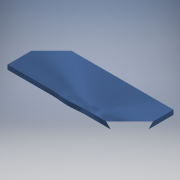
# Autodesk Inventor part: Cup_Dispenser_Slider_Cover
Saved by Autodesk Inventor 2016 (Build 200138000, 138)
## iProperties
Created: 2015-07-07
Part Number: Cup_Dispenser_Slider_Cover
Material: Generic
Document SubType Name: Modeling
Designer: 3DPrinterUser
Density: 1 g/cm^3
Appearance: Flaked Satin - Blue
Author: 3DPrinterUser
Autodesk Inventor part; units mm, degrees
ref_plane "YZ Plane" through (0, 0, 0) normal (1, 0, 0) x (0, 1, 0)
ref_plane "XZ Plane" through (0, 0, 0) normal (0, 1, 0) x (-1, 0, 0)
ref_plane "XY Plane" through (0, 0, 0) normal (0, 0, 1) x (1, 0, 0)
sketch "Sketch1" plane through (0, 0, 0) normal (0, 0, 1) x (1, 0, 0)
  line L0 (41, -16.75) -> (11.1915, -16.75) projected
  line L1 (41, -16.75) -> (41, -12.75) projected
  line L2 (-41, -12.75) -> (41, -12.75) projected
  line L3 (-41, -16.75) -> (-41, -12.75) projected
  line L4 (-11.1915, -16.75) -> (-41, -16.75) projected
  spline S0 degree 3 poles (-11.1915, -16.75) (-10.0304, -16.75) (-8.6395, -16.8333) (-6.313, -17.0219) (-5.0294, -17.1518) (-2.4598, -17.3597) (-1.173, -17.4271) (1.173, -17.4271) (2.4598, -17.3597) (5.0294, -17.1518) (6.313, -17.0219) (8.6395, -16.8333) (10.0304, -16.75) (11.1915, -16.75) knots 2.352794 2.352794 2.352794 2.352794 2.701135 2.701135 3.053026 3.053026 3.404917 3.404917 3.756807 3.756807 4.108698 4.108698 4.45704 4.45704 4.45704 4.45704 projected
  line L5 (-38, -6.75) -> (-38, 6.75) projected
  line L6 (-38, 6.75) -> (-36, 6.75) projected
  line L7 (-36, 6.75) -> (-36, 12.75) projected
  line L8 (-41, 12.75) -> (-36, 12.75) projected
  line L9 (-41, -12.75) -> (-41, 12.75) projected
  line L10 (-41, -12.75) -> (41, -12.75) projected
  line L11 (41, -12.75) -> (41, 12.75) projected
  line L12 (36, 12.75) -> (41, 12.75) projected
  line L13 (36, 6.75) -> (36, 12.75) projected
  line L14 (36, 6.75) -> (38, 6.75) projected
  line L15 (38, 6.75) -> (38, -6.75) projected
  line L16 (38, -6.75) -> (-38, -6.75) projected
  line L17 (36, 12.75) -> (-36, 12.75)
  point P0 (0, 0)
  constraints: 2 end point, 1 perpendicular
extrude "Extrusion1" add sketch "Sketch1" along normal blind 3
body "Solid1"
